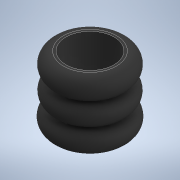
# Autodesk Inventor part: Air Suspension Air Bag
Saved by Autodesk Inventor 2022 (Build 260153000, 153)
## iProperties
Created: 2021-07-29
Part Number: Air Suspension Air Bag
Material: Rubber, Silicone
Document SubType Name: Modeling
Designer: WASHINGTON
Density: 1.25 g/cm^3
Appearance: Rubber - Black
Author: WASHINGTON
Autodesk Inventor part; units mm, degrees
ref_plane "YZ Plane" through (0, 0, 0) normal (1, 0, 0) x (0, 1, 0)
ref_plane "XZ Plane" through (0, 0, 0) normal (0, 1, 0) x (-1, 0, 0)
ref_plane "XY Plane" through (0, 0, 0) normal (0, 0, 1) x (1, 0, 0)
sketch "Sketch2" plane through (0, 0, 0) normal (0, 0, 1) x (1, 0, 0)
  point P0 (0, 0)
sketch "Sketch3" plane through (0, 0, 0) normal (0, 0, 1) x (1, 0, 0)
  line L0 (0, 0) -> (110, 0)
  line L1 (0, 0) -> (0, 141) construction
  line L2 (50, 141) -> (55, 141)
  arc A0 (55, 94) -> (55, 141) centre (54.2479, 117.5) ccw
  arc A1 (55, 47) -> (55, 94) centre (53.8712, 70.5) ccw
  arc A2 (55, 0) -> (55, 47) centre (55, 23.5) ccw
  line L3 (50, 141) -> (50, 0)
  dimension "d7" = 141
  dimension "d8" = 50
  dimension "d9" = 5
  dimension "d12" = 23.512
  dimension "d13" = 23.5271
  dimension "d14" = 23.5
  constraints: 8 end point, 6 point on circle, 3 centre point, 1 horizontal, 1 midpoint, 1 point on line, 1 vertical
  measures "d7" distance of L0.start L1.end
  measures "d8" distance of L1.end L2.start
  measures "d9" distance of L2.start L2.end
  measures "d12" radius of A0
  measures "d13" radius of A1
  measures "d14" radius of A2
revolve "Revolution1" add sketch "Sketch3" angle 360 about axis through (0, 0, 0) along (0, 1, 0)
body "Solid1"
